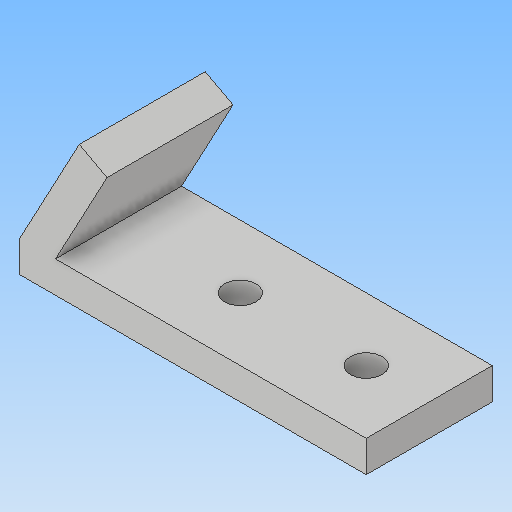
# Autodesk Inventor part: 防水5
Saved by Autodesk Inventor 2020 (Build 240168000, 168)
## iProperties
Part Number: 防水5
Material: 一般
Document SubType Name: Modeling
Designer: highs
Density: 1 g/cm^3
Appearance: 既定
Author: highs
## iProperties of the stored document 防水5_3D プリント.ipt
Part Number: 防水5_3D プリント
Material: 一般
Document SubType Name: Modeling
Designer: highs
Density: 1 g/cm^3
Appearance: 既定
Author: highs
Autodesk Inventor part; units mm, degrees
ref_plane "YZ Plane" through (0, 0, 0) normal (1, 0, 0) x (0, 1, 0)
ref_plane "XZ Plane" through (0, 0, 0) normal (0, 1, 0) x (-1, 0, 0)
ref_plane "XY Plane" through (0, 0, 0) normal (0, 0, 1) x (1, 0, 0)
sketch "スケッチ1" plane through (0, 0, 0) normal (0, 0, 1) x (1, 0, 0)
  line L0 (0, 0) -> (-55, 0)
  line L1 (-55, 0) -> (-55, 5)
  line L2 (-55, 5) -> (-45.5551, 22.6294)
  line L3 (-45.5551, 22.6294) -> (-41.1478, 20.2682)
  line L4 (-41.1478, 20.2682) -> (-49.3276, 5)
  line L5 (-49.3276, 5) -> (0, 5)
  line L6 (0, 5) -> (0, 0)
  dimension "d0" = 61.82
  dimension "d1" = 55
  dimension "d2" = 5
  dimension "d3" = 5
  dimension "d4" = 20
  constraints: 14 end point, 4 perpendicular, 1 horizontal, 1 parallel, 1 point on line
  measures "d0" angle of L0 L2
  measures "d1" distance of L0.start L0.end
  measures "d2" distance of L5.end L0.start
  measures "d3" distance between parallel lines of L2 L4
  measures "d4" distance of L1.end L2.end
extrude "押し出し1" add sketch "スケッチ1" along normal blind 20
sketch "スケッチ2" plane through (-55, 0, 0) normal (0, -1, 0) x (1, 0, 0)
  line L0 (55, 0) -> (55, 20) projected
  line L1 (55, 10) -> (45, 10) construction
  circle A0 centre (45, 10) radius 2.5
  circle A1 centre (25, 10) radius 2.5
  dimension "d7" = 5
  dimension "d8" = 10
  dimension "d11" = 20
  constraints: 2 centre point, 2 end point, 1 coincident, 1 equal radius, 1 horizontal, 1 midpoint, 1 point on line
  measures "d7" diameter of A0
  measures "d8" distance of L1.start L1.end
  measures "d11" distance of A0.centre A1.centre
extrude "押し出し2" cut sketch "スケッチ2" against normal up to next
